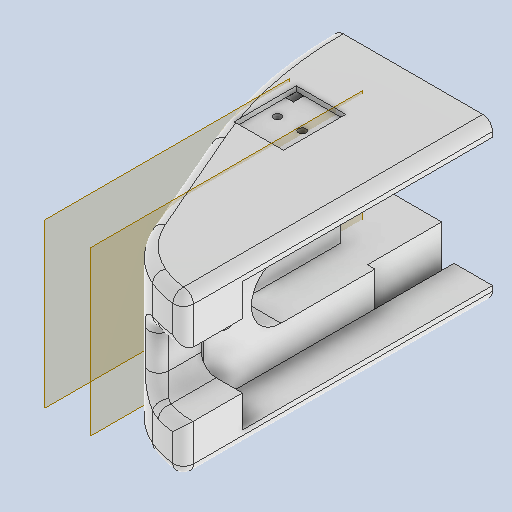
# Autodesk Inventor part: MontageAufnahmeLO
Saved by Autodesk Inventor 2025 (Build 290162010, 162A)
## iProperties
Created: 2024-11-18
Part Number: MontageAufnahmeLO
Material: PC/ABS-Kunststoff, 3DDruck, PLA
Document SubType Name: Modeling
Designer: Admin
Density: 1.1 g/cm^3
Appearance: Glatt - Weiß(2)
Mass: 29.2248 g
Surface Area: 64.7654 cm^2
Volume: 26.568 cm^3
Author: Admin
Autodesk Inventor part; units mm, degrees
ref_plane "YZ Plane" through (0, 0, 0) normal (1, 0, 0) x (0, 1, 0)
ref_plane "XZ Plane" through (0, 0, 0) normal (0, 1, 0) x (-1, 0, 0)
ref_plane "XY Plane" through (0, 0, 0) normal (0, 0, 1) x (1, 0, 0)
sketch "Skizze1" plane through (0, 0, 0) normal (0, 0, 1) x (1, 0, 0)
  line L0 (-9, -921.981078) -> (9, -921.981078)
  arc A0 (0.176471, -974.157548) -> (9, -982.981078) centre (15.747405, -967.410143) ccw
  line L1 (0.176471, -974.157548) -> (9, -974.157548) construction
  line L2 (9, -982.981078) -> (9, -974.157548)
  line L3 (9, -982.981078) -> (4, -982.981078) construction
  line L4 (9, -937.981078) -> (9, -974.157548)
  line L5 (-9, -952.981078) -> (0.176471, -974.157548)
  line L6 (7.5, -920.981078) -> (-7.5, -920.981078)
  line L7 (-7.5, -920.981078) -> (-7.5, -905.981078)
  line L8 (-7.5, -905.981078) -> (-9, -905.981078)
  line L9 (-9, -905.981078) -> (-9, -937.981078)
  line L10 (-9, -937.981078) -> (-7.5, -937.981078)
  line L11 (-7.5, -937.981078) -> (-7.5, -922.981078)
  line L12 (-7.5, -922.981078) -> (7.5, -922.981078)
  line L13 (7.5, -922.981078) -> (7.5, -937.981078)
  line L14 (7.5, -937.981078) -> (9, -937.981078)
  line L15 (9, -937.981078) -> (9, -905.981078)
  line L16 (9, -905.981078) -> (7.5, -905.981078)
  line L17 (7.5, -905.981078) -> (7.5, -920.981078)
  line L18 (-9, -937.981078) -> (-9, -952.981078)
  arc A1 (-15.427887, -921.981078) -> (-9, -952.981078) centre (62.538462, -921.981078) ccw
  line L19 (-15.427887, -921.981078) -> (-9, -921.981078)
  line L20 (-9, -921.981078) -> (-9, -937.981078)
  arc A2 (9, -982.981078) -> (16.8, -984.598417) centre (16.8, -964.981078) ccw
  line L21 (16.8, -984.598417) -> (16.8, -921.981078)
  line L22 (16.8, -921.981078) -> (9, -921.981078)
  line L23 (-9.05, -948.43137) -> (0.95, -948.43137)
  line L24 (-9.05, -935.83137) -> (-9.05, -948.43137)
  line L25 (0.95, -948.43137) -> (0.95, -935.83137)
  line L26 (0.95, -935.83137) -> (-9.05, -935.83137)
  line L27 (16.8, -972.598417) -> (9, -972.598417)
  line L28 (9, -972.598417) -> (8.5, -972.598417)
  line L29 (8.5, -972.598417) -> (8.5, -982.754738)
  point P0 (0, 0)
  dimension "d0" = 5
  dimension "d1" = 45
  dimension "d4" = 15
  dimension "d56" = 7.8
  dimension "d61" = 12
  dimension "d65" = 0.5
  constraints: 36 end point, 7 perpendicular, 7 point on circle, 5 vertical, 4 horizontal, 3 centre point, 3 point on line, 3 tangent, 2 line through centre, 2 midpoint, 1 coincident, 1 collinear, 4 other
  measures "d0" distance of L3.start L3.end
  measures "d1" distance of L4.start L3.start
  measures "d4" distance of L9.end L5.start
  measures "d56" distance between parallel lines of L21 L4
  measures "d61" distance from line of L27 L21.start
  measures "d65" distance of L27.end L28.end
extrude "Extrusion1" add sketch "Skizze1" against normal blind 30 contours L9 L26 L24 L23 L18 A1 L19 | L9 L18 L23 L24 L26 | L4 L28 L29 A0 L5 L18 L23 L25 L26 L11 L12 L13 L14 | L10 L11 L26 L25 L23 L18
sketch "Skizze3" plane through (0, 0, 0) normal (0, 0, 1) x (1, 0, 0)
  circle A0 centre (-13.05, -942.13137) radius 1.621 construction
  line L0 (-13.05, -942.13137) -> (-6.55, -942.13137) construction
  line L1 (-6.55, -942.13137) -> (-1.55, -942.13137) construction
  point P0 (0, 0)
  dimension "d14" = 6.5
  dimension "d15" = 5
  constraints: 4 coincident, 4 end point, 1 horizontal, 1 point on line
  measures "d14" distance of L0.start L0.end
  measures "d15" distance of L0.end L1.end
hole "Bohrung2" at (-6.55, -942.13137, 0) at (-1.55, -942.13137, 0) direction (0, 0, -1) diameter 1.567 depth 10 tip angle 118 thread size "M2x0.4" class "6H" standard "ANSI Metric M Profile"
sketch "Skizze7" plane through (-7.5, -937.981078, 0) normal (-1, 0, 0) x (0, 0, 1)
  line L0 (0, 15) -> (-30, 15) projected
  line L1 (-9, 15) -> (-21, 15)
  line L2 (-21, 15) -> (-21, 1)
  line L3 (-9, 1) -> (-9, 15)
  line L4 (-15, 15) -> (-15, 1)
  line L5 (-21, 1) -> (-15, 1)
  line L6 (-9, 1) -> (-15, 1)
  point P0 (0, 937.981078)
  point P1 (-9, 8)
  point P2 (-21, 15)
  dimension "d40" = 14
  dimension "d41" = 12
  constraints: 12 end point, 3 midpoint, 2 equal length, 2 horizontal, 1 collinear, 1 perpendicular, 1 point on line
  measures "d40" distance of L4.start L4.end
  measures "d41" distance from line of point (-9, 8) L2
extrude "Extrusion2" cut sketch "Skizze7" against normal through all
ref_plane "Arbeitsebene1" through (-1, -982.981078, 0) normal (1, 0, 0) x (0, 0, -1)
sketch "Skizze5" plane through (-1, -982.981078, 0) normal (1, 0, 0) x (0, 0, -1)
  line L0 (30, 45) -> (30, 10.382661)
  point P0 (0, 982.981078)
  point P1 (15, 15)
  point P2 (30, 0)
  dimension "d31" = 15
  dimension "d32" = 15
  measures "d31" distance from line of L0 point (15, 15)
  measures "d32" horizontal distance of point (30, 0) point (15, 15)
hole "Bohrung4" at (-1, -967.981078, -15) direction (1, 0, 0) diameter 3.2 end through all start extended yes countersink diameter 6.3 countersink angle 90 clearance for "Flachkopfmaschinenschraube" size "M3" standard "ANSI Metrisches M Profil"
sketch "Skizze9" plane through (9, -982.981078, 0) normal (1, 0, 0) x (0, 0, -1)
  circle A0 centre (15, 26) radius 6
  line L0 (21, 26) -> (21, 65.561839)
  line L1 (9, 26) -> (9, 65.561839)
  line L2 (9, 65.561839) -> (21, 65.561839)
  line L3 (0, 10.382661) -> (0, 45)
  line L4 (30, 45) -> (30, 10.382661)
  line L5 (0, 61) -> (30, 61)
  line L6 (15, 61) -> (15, 26)
  point P0 (0, 982.981078)
  dimension "d51" = 12
  dimension "d72" = 15
  dimension "d73" = 15
  dimension "d75" = 35
  constraints: 8 end point, 3 vertical, 2 horizontal, 2 point on circle, 2 tangent, 1 centre point, 1 midpoint
  measures "d51" diameter of A0
  measures "d72" distance from line of L3 L6.end
  measures "d73" distance from line of L4 L6.end
  measures "d75" distance from line of L5 L6.end
extrude "Extrusion3" cut sketch "Skizze9" against normal blind 8
ref_plane "Arbeitsebene2" through (-10.5, -982.981078, 0) normal (1, 0, 0) x (0, 0, -1)
sketch "Skizze8" plane through (-10.5, -952.981078, 0) normal (-1, 0, 0) x (0, 0, 1)
  line L0 (-15, 7.5) -> (-15, 0)
  line L1 (0, 0) -> (-30, 0) projected
  line L2 (0, 15) -> (-30, 15) projected
  line L3 (-15, 15) -> (-15, 7.5)
  point P0 (0, 952.981078)
  point P1 (-15, 3.75)
  constraints: 4 end point, 3 midpoint, 1 collinear, 1 perpendicular, 1 vertical
hole "Bohrung5" at (-10.5, -945.481078, -15) direction (1, 0, 0) diameter 3.2 end through all start extended yes countersink diameter 6.3 countersink angle 90 clearance for "Flachkopfmaschinenschraube" size "M3" standard "ANSI Metrisches M Profil"
extrude "Extrusion4" add sketch "Skizze1" along normal blind 1 contours L0 L15 L14 L13 L12 L11 L26 L9 | L9 L26 L24 L23 L18 A1 L19 | L22 L21 L27 L4 L15 | L4 L28 L29 A0 L5 L18 L23 L25 L26 L11 L12 L13 L14 | L27 L21 A2 L2 L4 | L4 L2 A0 L29 L28
extrude "Extrusion5" add sketch "Skizze1" against normal blind 2 contours L22 L21 L27 L4 L15 | L27 L21 A2 L2 L4 | L4 L2 A0 L29 L28
extrude "Extrusion6" add sketch "Skizze1" against normal blind 8.5 contours L27 L21 A2 L2 L4 | L4 L2 A0 L29 L28
fillet "Rundung2" radius 3 1 edges at (8.5, -977.6766, -8.5)
sketch "Skizze13" plane through (0, 0, -30) normal (0, 0, -1) x (-1, 0, 0)
  arc A0 (9, -952.981078) -> (15.427887, -921.981078) centre (-62.538462, -921.981078) ccw
  line L0 (-0.176471, -974.157548) -> (9, -952.981078)
  arc A1 (-16.8, -984.598417) -> (-9, -982.981078) centre (-16.8, -964.981078) ccw
  arc A2 (-9, -982.981078) -> (-0.176471, -974.157548) centre (-15.747405, -967.410143) ccw
  line L1 (15.427887, -921.981078) -> (9, -921.981078)
  line L2 (9, -921.981078) -> (9, -937.981078)
  line L3 (9, -937.981078) -> (7.5, -937.981078)
  line L4 (-7.5, -922.981078) -> (-7.5, -937.981078)
  line L5 (7.5, -922.981078) -> (-7.5, -922.981078)
  line L6 (7.5, -937.981078) -> (7.5, -922.981078)
  line L7 (-7.5, -937.981078) -> (-9, -937.981078)
  line L8 (-9, -937.981078) -> (-9, -921.981078)
  line L9 (-16.8, -984.598417) -> (-16.8, -921.981078)
  line L10 (-16.8, -921.981078) -> (-9, -921.981078)
  line L11 (-16.8, -972.598417) -> (-9, -972.598417)
  line L12 (-8.5, -972.598417) -> (-8.5, -982.754738)
  line L13 (-9, -972.598417) -> (-8.5, -972.598417)
  point P0 (0, 0)
  constraints: 6 end point, 2 vertical, 1 collinear, 1 perpendicular
extrude "Extrusion7" add sketch "Skizze13" along normal blind 1 and the other way blind 2
extrude "Extrusion8" add sketch "Skizze13" against normal blind 8.5 contours A2 A1 L9 L11 L13 L12
fillet "Rundung3" radius 3 1 edges at (8.5, -977.6766, -21.5)
fillet "Rundung4" radius 2 19 edges at (16.8, -953.2897, -31) (3.7478, -979.4098, -31) (-4.4118, -963.5693, -31) (-13.804, -937.8108, -31) (12.817, -984.1898, -31) (16.8, -984.5984, -26.25) (10.0053, -983.3841, -21.1011) (8.6248, -982.8131, -19.3562) (8.5, -982.7547, -15) (8.6248, -982.8131, -10.6438) (10.0056, -983.3842, -8.8987) (14.125, -984.4152, -8.5) (14.125, -984.4152, -21.5) (16.8, -984.5984, -3.75) (3.7478, -979.4098, 1) (-4.4118, -963.5693, 1) (-13.804, -937.8108, 1) (12.817, -984.1898, 1) (16.8, -953.2897, 1)
